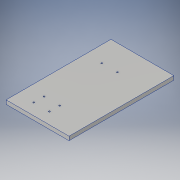
# Autodesk Inventor part: mplate03
Saved by Autodesk Inventor 2019 (Build 230136000, 136)
## iProperties
Created: 2022-09-05
Part Number: mplate03
Material: Aluminum 6061
Document SubType Name: Modeling
Designer: kananovicha
Density: 2.7 g/cm^3
Appearance: Aluminum - Flat
Author: kananovicha
Autodesk Inventor part; units mm, degrees
ref_plane "YZ Plane" through (0, 0, 0) normal (1, 0, 0) x (0, 1, 0)
ref_plane "XZ Plane" through (0, 0, 0) normal (0, 1, 0) x (-1, 0, 0)
ref_plane "XY Plane" through (0, 0, 0) normal (0, 0, 1) x (1, 0, 0)
sketch "Sketch1" plane through (0, 0, 0) normal (0, 0, 1) x (1, 0, 0)
  line L0 (-152.4, 9.525) -> (152.4, 9.525)
  line L1 (152.4, 9.525) -> (152.4, -9.525)
  line L2 (152.4, -9.525) -> (-152.4, -9.525)
  line L3 (-152.4, -9.525) -> (-152.4, 9.525)
  line L4 (-152.4, 9.525) -> (152.4, -9.525) construction
  line L5 (152.4, 9.525) -> (-152.4, -9.525) construction
  point P0 (0, 0)
  dimension "d0" = 304.8
  dimension "d1" = 19.05
  constraints: 12 end point, 2 midpoint, 2 parallel, 1 horizontal, 1 perpendicular
  measures "d0" distance of L1.end L2.end
  measures "d1" distance of L0.end L1.end
extrude "Extrusion1" add sketch "Sketch1" against normal blind 508
sketch "Sketch2" plane through (-152.4, 9.525, 0) normal (0, 1, 0) x (1, 0, 0)
  line L0 (0, 0) -> (0, 508) projected
  line L1 (0, 0) -> (304.8, 0) projected
  point P0 (152.4, 0)
  point P1 (78.245, 56)
  dimension "d4" = 78.245
  dimension "d5" = 56
  measures "d4" distance from line of point (78.245, 56) L0
  measures "d5" distance from line of point (78.245, 56) L1
hole "Hole1" at (-74.155, 9.525, -56) direction (0, -1, 0) diameter 6.9088 end through all
pattern_linear "Rectangular Pattern1" count 2 spacing 50 along (0, 0, -1) count 2 spacing 75.67 along (1, 0, 0) of "Hole1"
pattern_linear "Rectangular Pattern2" count 2 spacing 329.499 along (0, 0, -1) count 2 spacing 75.67 along (1, 0, 0) of "Hole1"
equation "\"d0\" = mp_wid"
equation "\"d1\" = mp_thick"
equation "\"d2\" = mp_len"
equation "\"d4\" = mp_mbra_holes_w_offset"
equation "\"d5\" = mp_mbra_holes_l_offset"
equation "\"d15\" = mp_mbra_holes_l_spacing"
equation "\"d18\" = mp_mbra_holes_w_spacing"
equation "\"d21\" = mp_bk_holes_distance"
equation "\"d24\" = mp_mbra_holes_w_spacing"
equation "\"mp_wid\" = 304.8"
equation "\"mp_thick\" = 19.05"
equation "\"mp_len\" = 508"
equation "\"mp_mbra_holes_l_spacing\" = 50"
equation "\"mp_mbra_holes_w_spacing\" = 75.67"
equation "\"mp_bk_holes_distance\" = 329.49896"
equation "\"mp_mbra_holes_w_offset\" = 78.245"
equation "\"mp_mbra_holes_l_offset\" = 56"
body "Solid1"
